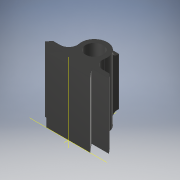
# Autodesk Inventor part: BT502_trajan20_21
Saved by Autodesk Inventor 2022.2 (Build 262287000, 287)
## iProperties
Company: HTBLA Kaindorf
RuleStatus: InUse
Created: 2022-08-09
Part Number: BT502_trajan20_21
Project: Zeichenmaschine_v2
Material: Kunststoff, undurchsichtig Schwarz
Description: Stifthalter innen
Document SubType Name: Modeling
Designer: trajan20
Density: 0.952 g/cm^3
Appearance: Glatt - Schwarz
Mass: 96.1701 g
Surface Area: 258.925 cm^2
Volume: 101.019 cm^3
AfterDocNew0: iProperties-Editor_aufrufen
Author: jan
Keywords: 2021
Autodesk Inventor part; units mm, degrees
ref_plane "YZ Plane" through (0, 0, 0) normal (1, 0, 0) x (0, 1, 0)
ref_plane "XZ Plane" through (0, 0, 0) normal (0, 1, 0) x (-1, 0, 0)
ref_plane "XY Plane" through (0, 0, 0) normal (0, 0, 1) x (1, 0, 0)
sketch "Skizze3" plane through (0, 0, 0) normal (0, 0, 1) x (1, 0, 0)
  line L0 (0, -25) -> (0, 25)
  line L1 (0, -25) -> (-10, -16.609)
  line L2 (0, 25) -> (-10, 16.609)
  line L3 (-10, -16.609) -> (-10, -36.609)
  line L4 (-10, 16.609) -> (-10, 36.609)
  circle A0 centre (-30, 0) radius 10
  line L5 (-54, 0) -> (9, 0) projected
  circle A1 centre (-30, 0) radius 15
  line L6 (-10, -36.609) -> (-15, -32.3721)
  line L7 (-10, 36.609) -> (-15, 32.3721)
  line L8 (-15, 32.3721) -> (-15, -32.3721)
  line L9 (-15, 5) -> (-15.8579, 5)
  line L10 (-15, -5) -> (-15.8579, -5)
  point P0 (0, 0)
  point P1 (0, 0)
  point P2 (-15, 0)
  dimension "d4" = 50
  dimension "d5" = 30
  dimension "d6" = 20
  dimension "d7" = 30
  dimension "d8" = 50
  dimension "d9" = 50
  dimension "d10" = 20
  dimension "d11" = 10
  dimension "d14" = 5
  constraints: 20 end point, 4 vertical, 3 point on line, 2 centre point, 2 coincident, 2 perpendicular, 2 point on circle, 2 tangent, 1 midpoint, 3 other
  measures "d4" distance of L0.start L0.end
  measures "d5" distance from line of L0 A0.centre
  measures "d6" diameter of A0
  measures "d7" diameter of A1
  measures "d8" angle of L3 L1
  measures "d9" angle of L4 L2
  measures "d10" distance of L1.end L3.end
  measures "d11" distance between parallel lines of L0 L3
  measures "d14" distance between parallel lines of L5 L10
extrude "Extrusion3" add sketch "Skizze3" along normal blind 75 contours L1 L3 L6 L8 L5 L0 | L5 L8 L7 L4 L2 L0 | A1 L5 A0 | L5 A0 A1 | L8 L10 A1 | A1 L9 L8
fillet "Rundung1" radius 10 4 edges at (-15, 5, 37.5) (-15.8579, 5, 37.5) (-15, -5, 37.5) (-15.8579, -5, 37.5)
ref_plane "Arbeitsebene2" through (-50, 0, 0) normal (1, 0, 0) x (0, 0, -1)
ref_plane "Arbeitsebene1" through (-45, 0, 0) normal (1, 0, 0) x (0, 0, -1)
sketch "Skizze5" plane through (-50, 0, 0) normal (1, 0, 0) x (0, 0, -1)
  line L0 (0, 15) -> (0, -15) projected
  line L1 (-75, 15) -> (-75, -15) projected
  line L2 (-10, -8) -> (-26, -8)
  line L3 (-26, -8) -> (-26, 8)
  line L4 (-26, 8) -> (-10, 8)
  line L5 (-10, 8) -> (-10, -8)
  line L6 (-49, -8) -> (-65, -8)
  line L7 (-65, -8) -> (-65, 8)
  line L8 (-65, 8) -> (-49, 8)
  line L9 (-49, 8) -> (-49, -8)
  line L10 (-75, 0) -> (0, 0) construction
  line L11 (-18, 8) -> (-18, -8) construction
  line L12 (-57, -8) -> (-57, 8) construction
  line L13 (-26, 8) -> (-49, 8)
  line L14 (-26, -8) -> (-49, -8)
  point P0 (0, 14.6969)
  point P1 (0, -14.6969)
  point P2 (-75, 14.6969)
  point P3 (-75, -14.6969)
  point P4 (-49, 0)
  point P5 (-26, 0)
  point P6 (-57, 0)
  point P7 (-18, 0)
  dimension "d18" = 10
  dimension "d19" = 16
  dimension "d21" = 10
  constraints: 26 end point, 8 midpoint, 7 perpendicular, 4 parallel, 4 point on line, 2 horizontal, 1 collinear, 1 vertical
  measures "d18" distance between parallel lines of L0 L5
  measures "d19" distance between parallel lines of L5 L3
  measures "d21" distance between parallel lines of L7 L1
extrude "Extrusion4" add sketch "Skizze5" along normal up to surface round surface about axis through (-30, 0, 0) along (0, 0, 1) radius 15 far side no
fillet "Rundung2" radius 5 2 edges at (-45, 0, 65) (-45, 0, 10)
hole "Bohrung1" at (-50, 0, 57) at (-50, 0, 18) direction (1, 0, 0) diameter 4.134 end up to face face through (-30, 0, 0) facing (0, 0, 1) round with radius 10 far side no thread size "M5x0.8" class "6H" standard "ISO Metric profile"
equation "\"d21\" = d18"
